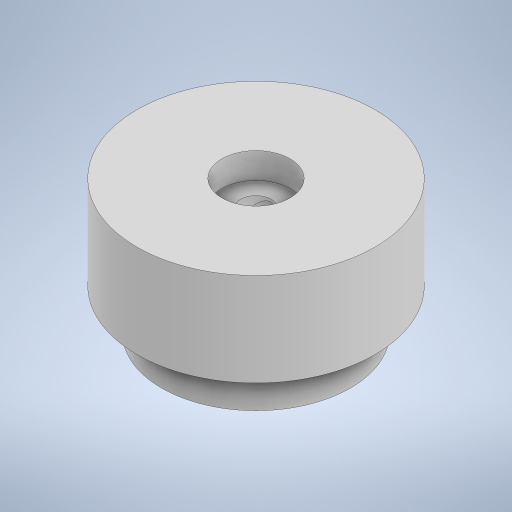
# Autodesk Inventor part: bottle
Saved by Autodesk Inventor 2023.1 (Build 271208000, 208)
## iProperties
Created: 2023-05-02
Part Number: bottle
Material: Generic
Document SubType Name: Modeling
Designer: dinesh
Density: 1 g/cm^3
Appearance: Default
Author: dinesh
Autodesk Inventor part; units mm, degrees
ref_plane "YZ Plane" through (0, 0, 0) normal (1, 0, 0) x (0, 1, 0)
ref_plane "XZ Plane" through (0, 0, 0) normal (0, 1, 0) x (-1, 0, 0)
ref_plane "XY Plane" through (0, 0, 0) normal (0, 0, 1) x (1, 0, 0)
sketch "Sketch1" plane through (0, 0, 0) normal (0, 0, 1) x (1, 0, 0)
  line L0 (3, 12) -> (23, 12)
  line L1 (23, 12) -> (23, 0)
  line L2 (3, 2) -> (3, 12)
  line L3 (0, 19.5472) -> (0, -22.4151)
  line L4 (23, 0) -> (22, 0) construction
  line L5 (22, 0) -> (22, -6)
  line L6 (22, -6) -> (23, -6)
  line L7 (23, -6) -> (23, 0)
  line L8 (20.4, 0) -> (17.25, 0) construction
  line L9 (17.25, 0) -> (17.25, -5) construction
  line L10 (17.25, -5) -> (20.4, -5) construction
  line L11 (20.4, -5) -> (20.4, 0)
  arc A0 (3, 2) -> (4.6637, 0.0285) centre (5, 2) ccw
  line L12 (22, 0) -> (20.4, 0)
  line L13 (17.25, 0) -> (5, 0)
  line L14 (-20.0393, 0) -> (22, 0) construction
  line L15 (23, 0) -> (24.5476, 0) construction
  line L16 (18.25, 0) -> (18.25, -5) construction
  line L17 (20.4, -5) -> (18.25, -5)
  line L18 (18.25, -5) -> (18.25, -14)
  line L19 (18.25, -14) -> (18.15, -14)
  line L20 (18.15, -14) -> (17.25, -5) construction
  line L21 (18.25, -8) -> (17.55, -8) construction
  line L22 (5.4025, -0.2566) -> (16.7316, -7.4783)
  line L23 (17.6466, -8.9658) -> (18.15, -14)
  arc A1 (17.6466, -8.9658) -> (16.7316, -7.4783) centre (15.6565, -9.1648) ccw
  arc A2 (5.4025, -0.2566) -> (4.6637, 0.0285) centre (4.3274, -1.943) ccw
  point P0 (0, 0)
  point P1 (17.25, 0)
  point P2 (17.25, -5)
  point P3 (5, 0)
  point P4 (17.9, -8)
  dimension "d0" = 6
  dimension "d2" = 1
  dimension "d5" = 5
  dimension "d6" = 1.6
  dimension "d7" = 44
  dimension "d11" = 2
  dimension "d12" = 12
  dimension "d14" = 6
  dimension "d23" = 36.5
  dimension "d24" = 1
  dimension "d25" = 0.1
  dimension "d26" = 9
  dimension "d37" = 3
  dimension "d38" = 2
  dimension "d39" = 2
  constraints: 48 end point, 14 point on line, 9 point on circle, 7 horizontal, 7 parallel, 6 collinear, 6 tangent, 5 perpendicular, 3 centre point, 3 vertical, 1 equal radius, 1 midpoint, 9 other
  measures "d0" diameter of L2 L3
  measures "d2" distance between parallel lines of L5 L7
  measures "d5" distance between parallel lines of L10 L8
  measures "d6" distance between parallel lines of L5 L11
  measures "d7" diameter of L5 L3
  measures "d11" radius of A0
  measures "d12" distance between parallel lines of L13 L0
  measures "d14" distance between parallel lines of L6 L4
  measures "d23" diameter of L16 L3
  measures "d25" distance of L18.end L19.end
  measures "d26" distance between parallel lines of L19 L10
  measures "d37" distance from line of point (17.9, -8) L10
  measures "d38" radius of A1
  measures "d39" radius of A2
revolve "Revolution1" add sketch "Sketch1" angle 360 about axis through (0, 19.5472, 0) along (0, -1, 0)
sketch "Sketch2" plane through (0, 0, 0) normal (0, 0, 1) x (1, 0, 0)
  line L0 (-3, 12) -> (3, 12) projected
  line L1 (0, 12) -> (0, 0) construction
  line L2 (-3, 2) -> (3, 2) construction
  circle A0 centre (0, 3.5) radius 3
  line L3 (-20.4, 0) -> (20.4, 0) projected
  point P0 (2.5981, 2)
  point P1 (-2.5981, 2)
  dimension "d16" = 6
  dimension "d40" = 3.5
  constraints: 2 end point, 1 centre point, 1 midpoint, 1 perpendicular, 1 point on line
  measures "d16" diameter of A0
  measures "d40" distance from line of L3 A0.centre
extrude "Extrusion1" cut sketch "Sketch2" along normal blind 3 and the other way blind 33
sketch "Sketch3" plane through (0, 12, 0) normal (0, 1, 0) x (1, 0, 0)
  circle A0 centre (0, 0) radius 6.575
  circle A1 centre (0, 0) radius 3 construction
  dimension "d27" = 13.15
  constraints: 1 centre point, 1 coincident, 1 concentric
  measures "d27" diameter of A0
extrude "Extrusion2" cut sketch "Sketch3" against normal blind 5
equation "\"d0\" = t_D"
equation "\"d2\" = w_th"
equation "\"d5\" = b_rim_h"
equation "\"d6\" = lv_th"
equation "\"d7\" = b_OD"
equation "\"d11\" = fillet_D"
equation "\"d12\" = top_th_f"
equation "\"d14\" = w_l"
equation "\"d23\" = b_ID"
equation "\"d24\" = w_th"
equation "\"d25\" = tol"
equation "\"d26\" = 1.5 * w_l"
equation "\"d37\" = 0.5 * w_l"
equation "\"d38\" = fillet_D"
equation "\"d39\" = fillet_D"
equation "\"d16\" = t_D"
equation "\"d40\" = 0.5 * w_th + 0.5 * t_D"
equation "\"d18\" = 0.5 * t_D"
equation "\"d19\" = 0.75 * b_OD"
equation "\"d27\" = cn_D"
equation "\"d30\" = cn_h"
equation "\"tol\" = 0.1"
equation "\"fillet_D\" = 2"
equation "\"w_th\" = 1"
equation "\"w_l\" = 6"
equation "\"t_D\" = 6"
equation "\"t_D_f\" = t_D + w_th"
equation "\"top_th_f\" = t_D_f + cn_h"
equation "\"cn_h\" = 5"
equation "\"lv_th\" = 1.6"
equation "\"d3\" = w_l"
equation "\"d8\" = top_th_f"
equation "\"b_ID\" = 36.5"
equation "\"b_OD\" = 44"
equation "\"b_rim_h\" = 5"
equation "\"top_th\" = t_D + w_th"
equation "\"lv_OD\" = 26"
equation "\"sv_OD\" = 13"
equation "\"sv_th\" = 1.5"
equation "\"b_th\" = 1.5"
equation "\"h_s\" = 2.25"
equation "\"h_D\" = 0.75"
equation "\"v_h_D\" = 7.5"
equation "\"v_h_off\" = 0.5 * cn_D + 0.5 * v_h_D"
equation "\"cn_D\" = 13.15"
body "Solid1"
